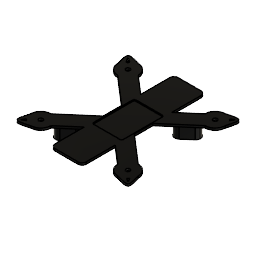
ICARUS 3 POLEGADAS CHASSI - DESATUALIZADO (Autodesk Fusion 360 design; units mm, degrees)
Autodesk Fusion 360 part; units mm, degrees
note: some values were not read from the file. Set by a fixed rule: which sketch regions a step uses.
sketch "Esboço1" plane through (0, 0, 0) normal (0, 0, 1) x (1, 0, 0)
  line L0 (14, -75) -> (-14, -75)
  line L1 (-19, -70) -> (-19, 70)
  line L2 (-14, 75) -> (14, 75)
  line L3 (19, 70) -> (19, -70)
  line L4 (19, -75) -> (-19, 75) construction
  line L5 (-19, -75) -> (19, 75) construction
  arc A0 (-14, 75) -> (-19, 70) centre (-14, 70) ccw
  arc A1 (19, 70) -> (14, 75) centre (14, 70) ccw
  arc A2 (14, -75) -> (19, -70) centre (14, -70) ccw
  arc A3 (-19, -70) -> (-14, -75) centre (-14, -70) ccw
  dimension "d1" = 38
  dimension "d2" = 150
  dimension "d3" = 5
  dimension "d4" = 5
  dimension "d5" = 5
  dimension "d6" = 5
  constraint horizontal L0
  constraint perpendicular L0 L1
  constraint parallel L0 L2
  constraint parallel L1 L3
  constraint coincident L4 origin
  constraint coincident L5 origin
  constraint coincident L4.end L2
  constraint coincident L4.end L1
  constraint tangent L2 A0
  constraint tangent L1 A0
  constraint coincident L5.end L2
  constraint coincident L5.end L3
  constraint tangent L2 A1
  constraint tangent L3 A1
  constraint coincident L4.start L0
  constraint coincident L4.start L3
  constraint tangent L0 A2
  constraint tangent L3 A2
  constraint coincident L5.start L0
  constraint coincident L5.start L1
  constraint tangent L0 A3
  constraint tangent L1 A3
  measures "d1" distance of L4.end L5.end
  measures "d2" distance of L5.start L4.end
  measures "d3" radius of A0
  measures "d4" radius of A1
  measures "d5" radius of A2
  measures "d6" radius of A3
extrude "Extrusão1" add sketch "Esboço1" along normal blind 2.5
sketch "Esboço2" plane through (0, 0, 2.5) normal (0, 0, 1) x (-1, 0, 0)
  arc A0 (14, -75) -> (19, -70) centre (14, -70) ccw
  line L0 (19, -70) -> (19, 70)
  arc A1 (19, 70) -> (14, 75) centre (14, 70) ccw
  line L1 (14, 75) -> (-14, 75)
  arc A2 (-14, 75) -> (-19, 70) centre (-14, 70) ccw
  line L2 (-19, 70) -> (-19, -70)
  arc A3 (-19, -70) -> (-14, -75) centre (-14, -70) ccw
  line L3 (-14, -75) -> (14, -75)
  line L4 (19, 0) -> (-19, 0) construction
  line L5 (16, 25.75) -> (-16, 25.75)
  line L6 (-18, 23.75) -> (-18, -23.75)
  line L7 (-16, -25.75) -> (16, -25.75)
  line L8 (18, -23.75) -> (18, 23.75)
  line L9 (18, 25.75) -> (-18, -25.75)
  line L10 (-18, 25.75) -> (18, -25.75)
  arc A4 (-16, 25.75) -> (-18, 23.75) centre (-16, 23.75) ccw
  arc A5 (18, 23.75) -> (16, 25.75) centre (16, 23.75) ccw
  arc A6 (16, -25.75) -> (18, -23.75) centre (16, -23.75) ccw
  arc A7 (-18, -23.75) -> (-16, -25.75) centre (-16, -23.75) ccw
  dimension "d9" = 36
  dimension "d10" = 51.5
  dimension "d74" = 2
  dimension "d75" = 2
  dimension "d76" = 2
  constraint midpoint L0 L4.start
  constraint midpoint L2 L4.end
  constraint horizontal L5
  constraint perpendicular L5 L6
  constraint parallel L5 L7
  constraint parallel L6 L8
  constraint coincident L9 origin
  constraint coincident L10 origin
  constraint coincident L10.start L5
  constraint coincident L10.start L6
  constraint tangent L5 A4
  constraint tangent L6 A4
  constraint coincident L9.start L8
  constraint coincident L9.start L5
  constraint tangent L8 A5
  constraint tangent L5 A5
  constraint coincident L10.end L7
  constraint coincident L10.end L8
  constraint tangent L7 A6
  constraint tangent L8 A6
  constraint equal A5 A6
  constraint coincident L9.end L7
  constraint coincident L9.end L6
  constraint tangent L7 A7
  constraint tangent L6 A7
  measures "d9" distance of L9.end L10.end
  measures "d10" distance of L10.start L9.end
  measures "d74" radius of A4
  measures "d75" radius of A5
  measures "d76" radius of A7
extrude "Extrusão2" cut sketch "Esboço2" against normal blind 1.5 contours L5 L9 L10 A4 A5 | L8 L9 L10 A5 A6 | L6 L9 L10 A4 A7 | L7 L9 L10 A6 A7
sketch "Esboço3" plane through (0, 0, 2.5) normal (0, 0, 1) x (-1, 0, 0)
  line L0 (-16, 25.75) -> (16, 25.75)
  line L1 (18, 23.75) -> (18, -23.75)
  line L2 (16, -25.75) -> (-16, -25.75)
  line L3 (-18, -23.75) -> (-18, 23.75)
  arc A0 (14, -75) -> (19, -70) centre (14, -70) ccw
  line L4 (19, -70) -> (19, 70)
  arc A1 (19, 70) -> (14, 75) centre (14, 70) ccw
  line L5 (14, 75) -> (-14, 75)
  arc A2 (-14, 75) -> (-19, 70) centre (-14, 70) ccw
  line L6 (-19, 70) -> (-19, -70)
  arc A3 (-19, -70) -> (-14, -75) centre (-14, -70) ccw
  line L7 (-14, -75) -> (14, -75)
  line L8 (19, 0) -> (19, -11.25) construction
  line L9 (19, 0) -> (19.7942, 11.2219) construction
  line L10 (19, -11.25) -> (-19, -11.25) construction
  line L11 (19.7942, 11.2219) -> (-19, 11.2219) construction
  line L12 (-1.8732, 1.767) -> (0, 0) construction
  line L13 (-53.1, 53.1) -> (53.1, 53.1) construction
  line L14 (53.1, 53.1) -> (53.1, -53.1) construction
  line L15 (53.1, -53.1) -> (-53.1, -53.1) construction
  line L16 (-53.1, -53.1) -> (-53.1, 53.1) construction
  line L17 (-53.1, 53.1) -> (53.1, -53.1) construction
  line L18 (53.1, 53.1) -> (-53.1, -53.1) construction
  circle A4 centre (53.1, -53.1) radius 12.5
  circle A5 centre (-53.1, -53.1) radius 12.5
  circle A6 centre (-53.1, 53.1) radius 12.5
  circle A7 centre (53.1, 53.1) radius 12.5
  line L19 (53.1, -40.6) -> (19, -11.25)
  line L20 (19, -11.25) -> (19, -70) construction
  line L21 (39.6446, -53.1) -> (40.6, -53.1) construction
  line L22 (40.6, -53.1) -> (19, -34.5088)
  line L23 (82.0691, 0) -> (-103.2974, 0) construction
  line L24 (0, -65.516) -> (0, 69.07) construction
  line L25 (40.6, 53.1) -> (19, 34.5088)
  line L26 (53.1, 40.6) -> (19, 11.25)
  line L27 (-53.1, -40.6) -> (-19, -11.25)
  line L28 (-39.6446, -53.1) -> (-40.6, -53.1) construction
  line L29 (-40.6, -53.1) -> (-19, -34.5088)
  line L30 (-53.1, 40.6) -> (-19, 11.25)
  line L31 (-40.6, 53.1) -> (-19, 34.5088)
  spline S0 degree 2 poles (65.6, -53.0754) (70.6231, -70.6231) (52.8232, -65.5969) knots 0 0 0 2.969399 2.969399 2.969399 weights 1 2.821651 1
  spline S1 degree 2 poles (62.2524, -59.9872) (66.3064, -66.2499) (60.2708, -62.2226) knots 0 0 0 1.233128 1.233128 1.233128 weights 1 4.892995 1
  line L32 (62.8537, -60.9176) -> (61.0529, -62.7437) construction
  arc A8 (62.2524, -59.9872) -> (60.2708, -62.2226) centre (61.2616, -61.1049) ccw
  circle A9 centre (53.1, -53.1) radius 2.5
  arc A10 (-60.2708, -62.2226) -> (-62.2524, -59.9872) centre (-61.2616, -61.1049) ccw
  spline S2 degree 2 poles (-62.2524, -59.9872) (-66.3064, -66.2499) (-60.2708, -62.2226) knots 0 0 0 1.233128 1.233128 1.233128 weights 1 4.892995 1
  spline S3 degree 2 poles (-65.6, -53.0754) (-70.6231, -70.6231) (-52.8232, -65.5969) knots 0 0 0 2.969399 2.969399 2.969399 weights 1 2.821651 1
  circle A11 centre (-53.1, -53.1) radius 2.5
  spline S4 degree 2 poles (65.6, 53.0754) (70.6231, 70.6231) (52.8232, 65.5969) knots 0 0 0 2.969399 2.969399 2.969399 weights 1 2.821651 1
  spline S5 degree 2 poles (62.2524, 59.9872) (66.3064, 66.2499) (60.2708, 62.2226) knots 0 0 0 1.233128 1.233128 1.233128 weights 1 4.892995 1
  arc A12 (60.2708, 62.2226) -> (62.2524, 59.9872) centre (61.2616, 61.1049) ccw
  circle A13 centre (53.1, 53.1) radius 2.5
  circle A14 centre (-53.1, 53.1) radius 2.5
  spline S6 degree 2 poles (-62.2524, 59.9872) (-66.3064, 66.2499) (-60.2708, 62.2226) knots 0 0 0 1.233128 1.233128 1.233128 weights 1 4.892995 1
  arc A15 (-62.2524, 59.9872) -> (-60.2708, 62.2226) centre (-61.2616, 61.1049) ccw
  spline S7 degree 2 poles (-65.6, 53.0754) (-70.6231, 70.6231) (-52.8232, 65.5969) knots 0 0 0 2.969399 2.969399 2.969399 weights 1 2.821651 1
  arc A16 (-18, -23.75) -> (-16, -25.75) centre (-16, -23.75) ccw
  arc A17 (-16, 25.75) -> (-18, 23.75) centre (-16, 23.75) ccw
  arc A18 (18, 23.75) -> (16, 25.75) centre (16, 23.75) ccw
  arc A19 (16, -25.75) -> (18, -23.75) centre (16, -23.75) ccw
  dimension "d13" = 11.25
  dimension "d14" = 11.25
  dimension "d41" = 106.2
  dimension "d42" = 106.2
  dimension "d43" = 25
  dimension "d44" = 25
  dimension "d45" = 25
  dimension "d46" = 25
  dimension "d67" = 5
  constraint midpoint L4 L8.start
  constraint coincident L6 L10.end
  constraint perpendicular L6 L10
  constraint coincident L6 L11.end
  constraint perpendicular L6 L11
  constraint coincident L12.end origin
  constraint horizontal L13
  constraint perpendicular L13 L14
  constraint parallel L13 L15
  constraint parallel L14 L16
  constraint coincident L17 L12.end
  constraint coincident L18 L12.end
  constraint coincident L14.end L15.start
  constraint coincident L15.end L16.start
  constraint coincident L13.start L16.end
  constraint coincident L13.end L14.start
  constraint coincident A4 L19.start
  constraint coincident L14 L19.start
  constraint coincident A0.end L4.start
  constraint tangent A0 L20
  constraint coincident L15 L21.start
  constraint coincident A4 L21.end
  constraint coincident L15 L21.end
  constraint coincident L20 L22.end
  constraint parallel L19 L22
  constraint perpendicular L1 L23
  constraint perpendicular L23 L24
  constraint symmetric L8.end L23 L26.end
  constraint symmetric L19.start L23 L26.start
  constraint symmetric L21.end L23 L25.start
  constraint symmetric L22.end L23 L25.end
  constraint symmetric L8.end L24 L10.end
  constraint symmetric L19.start L24 L27.start
  constraint symmetric L21.start L24 L28.start
  constraint symmetric L21.end L24 L28.end
  constraint symmetric L22.end L24 L29.end
  constraint symmetric L24 L25.start L31.start
  constraint symmetric L24 L25.end L31.end
  constraint symmetric L24 L26.start L30.start
  constraint symmetric L24 L26.end L30.end
  constraint coincident A4 S0.end
  constraint coincident A4 S0.start
  constraint coincident S1 L32.start
  constraint coincident A4 L32.start
  constraint coincident S1 L32.end
  constraint coincident A4 L32.end
  constraint concentric A4 A9
  constraint symmetric L24 S0.end S3.end
  constraint symmetric L24 S0.start S3.start
  constraint symmetric L24 S0 S3
  constraint symmetric L24 S1.start A10.end
  constraint symmetric L24 S1.end A10.start
  constraint symmetric L24 S1 S2
  constraint symmetric L24 A8 A10
  constraint symmetric L24 A9 A11
  constraint symmetric L23 S0.end S4.end
  constraint symmetric L23 S0.start S4.start
  constraint symmetric L23 S0 S4
  constraint symmetric L23 S1.start S5.start
  constraint symmetric L23 S1.end S5.end
  constraint symmetric L23 S1 S5
  constraint symmetric L23 A8 A12
  constraint symmetric L23 A9 A13
  constraint symmetric L23 A10.end S6.start
  constraint symmetric L23 A10.start S6.end
  constraint symmetric L23 A10 A15
  constraint symmetric L23 S2 S6
  constraint symmetric L23 S3.start S7.start
  constraint symmetric L23 S3.end S7.end
  constraint symmetric L23 S3 S7
  constraint symmetric L23 A11 A14
  measures "d13" distance of L8.start L8.end
  measures "d14" distance of L8.start L9.end
  measures "d41" distance of L14.end L15.end
  measures "d42" distance of L13.end L14.end
  measures "d43" diameter of A4
  measures "d44" diameter of A5
  measures "d45" diameter of A6
  measures "d46" diameter of A7
  measures "d67" diameter of A9
extrude "Extrusão3" add sketch "Esboço3" against normal blind 2.5 contours L4 A4 L19 L22 | A4 S1 A8 | L6 A5 L27 L29 | L4 A7 L25 L26 | A4 S0 S1 | A5 A10 S2 | A7 S5 A12 | L6 A6 L30 L31 | A5 S2 S3 | A7 S4 S5 | A6 S6 A15 | A5 A10 S2 | A6 S6 S7 | A7 S5 A12 | A6 S6 A15 picked at (56.5902, -60.5787)
sketch "Esboço4" plane through (0, 0, 0) normal (0, 0, -1) x (1, 0, 0)
  spline S0 degree 2 poles (61.0529, 62.7437) (66.272, 66.216) (62.8537, 60.9176) knots -1.214656 -1.214656 -1.214656 -0.021592 -0.021592 -0.021592 weights 1.114883 4.768557 1.133943
  arc A0 (62.8537, 60.9176) -> (61.0529, 62.7437) centre (53.1, 53.1) ccw
  circle A1 centre (53.1, 53.1) radius 2.5
  spline S1 degree 2 poles (-62.8537, 60.9176) (-66.272, 66.216) (-61.0529, 62.7437) knots 0.021592 0.021592 0.021592 1.214656 1.214656 1.214656 weights 1.133943 4.768557 1.114883
  arc A2 (-61.0529, 62.7437) -> (-62.8537, 60.9176) centre (-53.1, 53.1) ccw
  circle A3 centre (-53.1, 53.1) radius 2.5
  circle A4 centre (53.1, -53.1) radius 2.5
  spline S2 degree 2 poles (62.8537, -60.9176) (66.272, -66.216) (61.0529, -62.7437) knots 0.021592 0.021592 0.021592 1.214656 1.214656 1.214656 weights 1.133943 4.768557 1.114883
  arc A5 (61.0529, -62.7437) -> (62.8537, -60.9176) centre (53.1, -53.1) ccw
  arc A6 (-60.2708, -62.2226) -> (-62.2524, -59.9872) centre (-61.2616, -61.1049) ccw
  spline S3 degree 2 poles (-60.2708, -62.2226) (-66.3064, -66.2499) (-62.2524, -59.9872) knots -1.233128 -1.233128 -1.233128 0 0 0 weights 1 4.892995 1
  circle A7 centre (-53.1, -53.1) radius 2.5
  arc A8 (-19, -70) -> (-14, -75) centre (-14, -70) ccw
  line L0 (-14, -75) -> (14, -75)
  arc A9 (14, -75) -> (19, -70) centre (14, -70) ccw
  line L1 (19, -70) -> (19, -34.5088)
  line L2 (19, -34.5088) -> (40.6, -53.1)
  arc A10 (40.6, -53.1) -> (52.8232, -65.5969) centre (53.1, -53.1) ccw
  spline S4 degree 2 poles (52.8232, -65.5969) (70.6231, -70.6231) (65.6, -53.0754) knots -2.969399 -2.969399 -2.969399 0 0 0 weights 1 2.821651 1
  arc A11 (65.6, -53.0754) -> (53.1, -40.6) centre (53.1, -53.1) ccw
  line L3 (53.1, -40.6) -> (19, -11.25)
  line L4 (19, -11.25) -> (19, 11.25)
  line L5 (19, 11.25) -> (53.1, 40.6)
  arc A12 (53.1, 40.6) -> (65.6, 53.0754) centre (53.1, 53.1) ccw
  spline S5 degree 2 poles (65.6, 53.0754) (70.6231, 70.6231) (52.8232, 65.5969) knots 0 0 0 2.969399 2.969399 2.969399 weights 1 2.821651 1
  arc A13 (52.8232, 65.5969) -> (40.6, 53.1) centre (53.1, 53.1) ccw
  line L6 (40.6, 53.1) -> (19, 34.5088)
  line L7 (19, 34.5088) -> (19, 70)
  arc A14 (19, 70) -> (14, 75) centre (14, 70) ccw
  line L8 (14, 75) -> (-14, 75)
  arc A15 (-14, 75) -> (-19, 70) centre (-14, 70) ccw
  line L9 (-19, 70) -> (-19, 34.5088)
  line L10 (-19, 34.5088) -> (-40.6, 53.1)
  arc A16 (-40.6, 53.1) -> (-52.8232, 65.5969) centre (-53.1, 53.1) ccw
  spline S6 degree 2 poles (-52.8232, 65.5969) (-70.6231, 70.6231) (-65.6, 53.0754) knots -2.969399 -2.969399 -2.969399 0 0 0 weights 1 2.821651 1
  arc A17 (-65.6, 53.0754) -> (-53.1, 40.6) centre (-53.1, 53.1) ccw
  line L11 (-53.1, 40.6) -> (-19, 11.25)
  line L12 (-19, 11.25) -> (-19, -11.25)
  line L13 (-19, -11.25) -> (-53.1, -40.6)
  arc A18 (-53.1, -40.6) -> (-65.6, -53.0754) centre (-53.1, -53.1) ccw
  spline S7 degree 2 poles (-65.6, -53.0754) (-70.6231, -70.6231) (-52.8232, -65.5969) knots 0 0 0 2.969399 2.969399 2.969399 weights 1 2.821651 1
  arc A19 (-52.8232, -65.5969) -> (-40.6, -53.1) centre (-53.1, -53.1) ccw
  line L14 (-40.6, -53.1) -> (-19, -34.5088)
  line L15 (-19, -34.5088) -> (-19, -70)
  line L16 (19, 0) -> (-19, 0) construction
  line L17 (53.1, -40.6) -> (40.6, -53.1) construction
  line L18 (19, -34.5088) -> (40.6, -53.1) construction
  line L19 (19, -11.25) -> (19, -34.5088) construction
  line L20 (19, -11.25) -> (53.1, -40.6) construction
  line L21 (0, -75) -> (0, 75) construction
  line L22 (53.1, 0) -> (-49.7297, 0) construction
  line L23 (19, 11.25) -> (53.1, 40.6) construction
  line L24 (53.1, 40.6) -> (40.6, 53.1) construction
  line L25 (19, 34.5088) -> (40.6, 53.1) construction
  line L26 (19, 11.25) -> (19, 34.5088) construction
  line L27 (-19, 11.25) -> (-19, 34.5088) construction
  line L28 (-19, 34.5088) -> (-40.6, 53.1) construction
  line L29 (-19, 11.25) -> (-53.1, 40.6) construction
  line L30 (-53.1, 40.6) -> (-40.6, 53.1) construction
  line L31 (-19, -11.25) -> (-53.1, -40.6) construction
  line L32 (-53.1, -40.6) -> (-40.6, -53.1) construction
  line L33 (-19, -34.5088) -> (-40.6, -53.1) construction
  line L34 (-19, -11.25) -> (-19, -34.5088) construction
  line L35 (29.8, -43.8044) -> (41.2998, -30.4435) construction
  line L36 (36.05, -25.925) -> (24.5502, -39.2859) construction
  line L37 (35.5499, -37.124) -> (30.3001, -32.6054) construction
  line L38 (19, -22.8794) -> (46.85, -46.85) construction
  line L39 (44.6888, -37.124) -> (34.1892, -28.0869)
  arc A20 (34.1892, -28.0869) -> (26.411, -37.124) centre (30.3001, -32.6054) ccw
  line L40 (26.411, -37.124) -> (36.9106, -46.161)
  arc A21 (36.9106, -46.161) -> (44.6888, -37.124) centre (40.7997, -41.6425) ccw
  line L41 (40.7997, -41.6425) -> (30.3001, -32.6054) construction
  arc A22 (-44.6888, -37.124) -> (-36.9106, -46.161) centre (-40.7997, -41.6425) ccw
  line L42 (-26.411, -37.124) -> (-36.9106, -46.161)
  arc A23 (-26.411, -37.124) -> (-34.1892, -28.0869) centre (-30.3001, -32.6054) ccw
  line L43 (-44.6888, -37.124) -> (-34.1892, -28.0869)
  line L44 (26.411, 37.124) -> (36.9106, 46.161)
  arc A24 (44.6888, 37.124) -> (36.9106, 46.161) centre (40.7997, 41.6425) ccw
  line L45 (44.6888, 37.124) -> (34.1892, 28.0869)
  arc A25 (26.411, 37.124) -> (34.1892, 28.0869) centre (30.3001, 32.6054) ccw
  line L46 (-26.411, 37.124) -> (-36.9106, 46.161)
  arc A26 (-34.1892, 28.0869) -> (-26.411, 37.124) centre (-30.3001, 32.6054) ccw
  line L47 (-44.6888, 37.124) -> (-34.1892, 28.0869)
  arc A27 (-36.9106, 46.161) -> (-44.6888, 37.124) centre (-40.7997, 41.6425) ccw
  point P0 (35.5499, -37.124)
  constraint midpoint L4 L16.start
  constraint midpoint L12 L16.end
  constraint coincident A11.end L3.start
  constraint coincident L2.end A10.start
  constraint coincident L1.end L2.start
  constraint coincident L3.end L4.start
  constraint midpoint L0 L21.start
  constraint midpoint L8 L21.end
  constraint perpendicular L12 L22
  constraint symmetric A11.end L22 L5.end
  constraint symmetric L2.end L22 A13.end
  constraint symmetric L1.end L22 L6.end
  constraint symmetric L3.end L22 L4.end
  constraint symmetric A11.end L21 L13.end
  constraint symmetric L2.end L21 A19.end
  constraint symmetric L1.end L21 L14.end
  constraint symmetric L3.end L21 L12.end
  constraint symmetric L21 L4.end L11.end
  constraint symmetric L21 L5.end A17.end
  constraint symmetric L21 A13.end L10.end
  constraint symmetric L21 L6.end L9.end
  constraint midpoint L18 L35.start
  constraint coincident L20 L35.end
  constraint perpendicular L20 L35
  constraint midpoint L20 L36.start
  constraint coincident L18 L36.end
  constraint perpendicular L18 L36
  constraint midpoint L35 P0
  constraint midpoint L36 L37.end
  constraint midpoint L19 L38.start
  constraint midpoint L17 L38.end
  constraint tangent L39 A20
  constraint tangent A20 L40
  constraint parallel L39 L40
  constraint tangent L40 A21
  constraint tangent L39 A21
  constraint coincident L37.end A20.centre
  constraint perpendicular L36 L41
  constraint coincident P0 L37.start
  constraint midpoint L41 P0
  constraint symmetric L21 L39.start A22.start
  constraint symmetric L21 L39.end A23.end
  constraint symmetric L21 A20.end L42.start
  constraint symmetric L21 L40.end A22.end
  constraint symmetric L21 A20 A23
  constraint symmetric L21 A21 A22
  constraint symmetric L22 L39.start A24.start
  constraint symmetric L22 L39.end L45.end
  constraint symmetric L22 A20.end L44.start
  constraint symmetric L22 L40.end L44.end
  constraint symmetric L22 A20 A25
  constraint symmetric L22 A21 A24
  constraint symmetric L22 A22.end L46.end
  constraint symmetric L22 A22.start L47.start
  constraint symmetric L22 A22 A27
  constraint symmetric L22 L42.start L46.start
  constraint symmetric L22 A23.end A26.start
  constraint symmetric L22 A23 A26
extrude "Extrusão4" add sketch "Esboço4" along normal blind 15 contours L39 A20 L40 A21 | A22 L42 A23 L43 | L44 A24 L45 A25 | L46 A26 L47 A27
equation "d64 = 0.738333"
equation "d66 = 0.830307"
equation "d68 = d66"
equation "d69 = d64"
equation "d70 = d64"
equation "d71 = d66"
equation "d72 = d68"
equation "d73 = d69"
